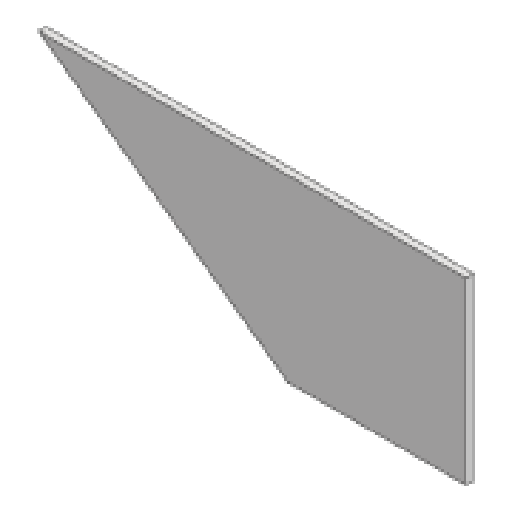
# Autodesk Inventor part: frontLeftSidePlateV2
Saved by Autodesk Inventor 2025 (Build 290162000, 162)
## iProperties
Created: 2025-01-06
Part Number: frontLeftSidePlateV2
Material: Generic
Document SubType Name: Modeling
Designer: derm
Density: 1 g/cm^3
Appearance: Default
Author: derm
Autodesk Inventor part; units mm, degrees
ref_plane "YZ Plane" through (0, 0, 0) normal (1, 0, 0) x (0, 1, 0)
ref_plane "XZ Plane" through (0, 0, 0) normal (0, 1, 0) x (-1, 0, 0)
ref_plane "XY Plane" through (0, 0, 0) normal (0, 0, 1) x (1, 0, 0)
sketch "Sketch1" plane through (0, 0, 0) normal (0, 0, 1) x (1, 0, 0)
  line L0 (0, 0) -> (-166.8883, 119.871)
  line L1 (-166.8883, 119.871) -> (118.9149, 119.871)
  line L2 (118.9149, 119.871) -> (118.9149, 0)
  line L3 (118.9149, 0) -> (0, 0)
  line L4 (385.7085, 119.871) -> (-223.8915, 119.871) projected
  line L5 (-0.2224, 6.0906) -> (-134.4097, 122.7379) projected
  line L6 (159.6989, 0) -> (330.9455, 0) projected
  line L7 (-119.1192, 85.4511) -> (-192.965, 138.6604) projected
  constraints: 8 end point, 2 perpendicular, 2 point on line, 1 horizontal
extrude "Extrusion1" add sketch "Sketch1" against normal blind 5
body "Solid1"
